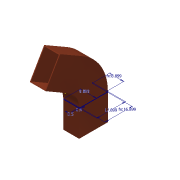
# Autodesk Inventor part: curved waveguide120
Saved by Autodesk Inventor 2015 (Build 190159000, 159)
## iProperties
Created: 2014-05-19
Part Number: curved waveguide120
Material: Generic
Document SubType Name: Modeling
Designer: jad211
Density: 1 g/cm^3
Appearance: Copper - Satin
Author: jad211
Autodesk Inventor part; units mm, degrees
ref_plane "YZ Plane" through (0, 0, 0) normal (1, 0, 0) x (0, 1, 0)
ref_plane "XZ Plane" through (0, 0, 0) normal (0, 1, 0) x (-1, 0, 0)
ref_plane "XY Plane" through (0, 0, 0) normal (0, 0, 1) x (1, 0, 0)
sketch "Sketch1" plane through (0, 0, 0) normal (0, 1, 0) x (-1, 0, 0)
  line L0 (0, 0) -> (9.899, 0)
  line L1 (9.899, 0) -> (9.899, -17.899)
  line L2 (9.899, -17.899) -> (0, -17.899)
  line L3 (0, -17.899) -> (0, 0)
  line L4 (0.5, -0.5) -> (9.399, -0.5)
  line L5 (9.399, -0.5) -> (9.399, -17.399)
  line L6 (9.399, -17.399) -> (0.5, -17.399)
  line L7 (0.5, -17.399) -> (0.5, -0.5)
  dimension "d0" = 9.899
  dimension "d1" = 17.899
  dimension "d2" = 16.899
  dimension "d3" = 8.899
  dimension "d4" = 0.5
  dimension "d5" = 0.5
  constraints: 16 end point, 4 parallel, 2 horizontal, 2 perpendicular
  measures "d0" distance of L0.start L0.end
  measures "d1" distance of L0.end L1.end
  measures "d2" distance of L4.end L5.end
  measures "d3" distance of L5.end L6.end
  measures "d4" distance between parallel lines of L7 L3
  measures "d5" distance between parallel lines of L0 L4
sketch "Sketch3" plane through (0, 0, 0) normal (1, 0, 0) x (0, 1, 0)
  arc A0 (0, 0) -> (11.2583, 6.5) centre (0, 13) ccw
  line L0 (0, 13) -> (11.2583, 6.5) construction
  line L1 (0, 13) -> (0, 0) construction
  dimension "d6" = 60
  dimension "d7" = 13
  constraints: 4 end point, 2 point on circle, 1 centre point
  measures "d6" angle of L1 L0
  measures "d7" distance of L1.end L0.start
sweep "Sweep1" add profiles "Sketch1" path "Sketch3"
extrude "Extrusion1" add sketch "Sketch1" against normal blind 16.55
ref_plane "Work Plane1" through (-9.899, 11.2583, 6.5) normal (0, 0.5, 0.866) x (1, 0, 0)
sketch "Sketch4" plane through (-9.899, 11.2583, 6.5) normal (0, 0.5, 0.866) x (1, 0, 0)
  line L0 (0, 0) -> (9.899, 0)
  line L1 (0, 0) -> (0, 17.899)
  line L2 (0, 17.899) -> (9.899, 17.899)
  line L3 (9.899, 17.899) -> (9.899, 0)
  line L4 (0.5, 17.399) -> (9.399, 17.399)
  line L5 (9.399, 17.399) -> (9.399, 0.5)
  line L6 (9.399, 0.5) -> (0.5, 0.5)
  line L7 (9.399, 0.5) -> (0.5, 0.5) projected
  line L8 (0.5, 0.5) -> (0.5, 17.399)
  constraints: 16 end point, 4 perpendicular, 2 horizontal, 1 collinear, 1 vertical
extrude "Extrusion2" add sketch "Sketch4" along normal blind 16.55
body "Solid1"
